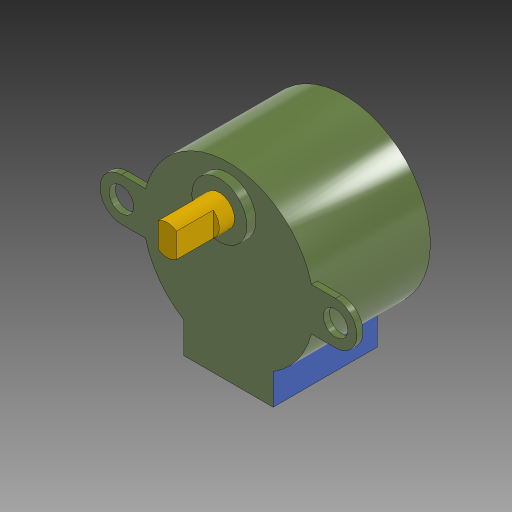
# Autodesk Inventor part: StepperMotor
Saved by Autodesk Inventor 2023 (Build 270158000, 158)
## iProperties
Created: 2024-02-02
Part Number: StepperMotor
Material: Všeobecné
Document SubType Name: Modeling
Designer: matej
Mass: 12.9017 g
Surface Area: 35.146 cm^2
Volume: 12.9017 cm^3
Density: 1 g/cm^3
Appearance: Tmavě olivová
Author: matej
Autodesk Inventor part; units mm, degrees
ref_plane "YZ Plane" through (0, 0, 0) normal (1, 0, 0) x (0, 1, 0)
ref_plane "XZ Plane" through (0, 0, 0) normal (0, 1, 0) x (-1, 0, 0)
ref_plane "XY Plane" through (0, 0, 0) normal (0, 0, 1) x (1, 0, 0)
sketch "Náčrt1" plane through (0, 0, 0) normal (0, 0, 1) x (1, 0, 0)
  circle A0 centre (0, 0) radius 14
  dimension "d0" = 28
  constraints: 1 centre point, 1 coincident
  measures "d0" diameter of A0
extrude "Vysunutí1" add sketch "Náčrt1" along normal blind 19
sketch "Náčrt2" plane through (0, 0, 19) normal (0, 0, 1) x (1, 0, 0)
  circle A0 centre (17.5, 0) radius 2
  circle A1 centre (-17.5, 0) radius 2
  line L0 (-17.5, 0) -> (17.5, 0) construction
  line L1 (-17.5, -3.5) -> (17.5, -3.5)
  line L2 (17.5, 3.5) -> (-17.5, 3.5)
  arc A2 (-17.5, 3.5) -> (-17.5, -3.5) centre (-17.5, 0) ccw
  arc A3 (17.5, -3.5) -> (17.5, 3.5) centre (17.5, 0) ccw
  point P0 (0, 0)
  point P1 (0, 0)
  dimension "d3" = 4
  dimension "d4" = 4
  dimension "d5" = 35
  dimension "d9" = 17.5
  dimension "d10" = 7
  constraints: 8 end point, 4 centre point, 4 point on circle, 4 tangent, 1 horizontal, 1 midpoint, 1 parallel
  measures "d3" diameter of A0
  measures "d4" diameter of A1
  measures "d5" distance of L0.end L0.start
  measures "d9" distance of point (0, 0) L0.end
  measures "d10" diameter of A3
extrude "Vysunutí2" add sketch "Náčrt2" against normal blind 1
sketch "Náčrt3" plane through (0, 0, 19) normal (0, 0, 1) x (1, 0, 0)
  circle A0 centre (0, 8) radius 4.5
  point P0 (0, 0)
  dimension "d13" = 9
  dimension "d14" = 8
  constraints: 1 centre point
  measures "d13" diameter of A0
  measures "d14" distance of point (0, 0) A0.centre
extrude "Vysunutí3" add sketch "Náčrt3" along normal blind 1.5
sketch "Náčrt4" plane through (0, 8, 20.5) normal (0, 0, 1) x (1, 0, 0)
  circle A0 centre (0, 0) radius 2.5
  point P0 (0, -8)
  dimension "d17" = 5
  constraints: 1 centre point
  measures "d17" diameter of A0
extrude "Vysunutí4" add sketch "Náčrt4" along normal blind 8.5
sketch "Náčrt5" plane through (0, 8, 29) normal (0, 0, 1) x (1, 0, 0)
  line L0 (-1.5, -2.5) -> (1.5, -2.5)
  line L1 (1.5, -2.5) -> (1.5, 2.5)
  line L2 (1.5, 2.5) -> (-1.5, 2.5)
  line L3 (-1.5, 2.5) -> (-1.5, -2.5)
  line L4 (-1.5, -2.5) -> (1.5, 2.5) construction
  line L5 (1.5, -2.5) -> (-1.5, 2.5) construction
  line L6 (-3, -3) -> (3, -3)
  line L7 (3, -3) -> (3, 3)
  line L8 (3, 3) -> (-3, 3)
  line L9 (-3, 3) -> (-3, -3)
  line L10 (-3, -3) -> (3, 3) construction
  line L11 (3, -3) -> (-3, 3) construction
  point P0 (0, -8)
  point P1 (0, 0)
  point P2 (0, 0)
  dimension "d20" = 3
  dimension "d21" = 5
  dimension "d22" = 6
  dimension "d23" = 6
  constraints: 24 end point, 5 midpoint, 4 parallel, 2 horizontal, 2 perpendicular
  measures "d20" distance of L2.end L1.end
  measures "d21" distance of L1.end L0.end
  measures "d22" distance of L8.end L7.end
  measures "d23" distance of L7.end L6.end
extrude "Vysunutí5" cut sketch "Náčrt5" against normal blind 6
sketch "Náčrt6" plane through (0, 0, 19) normal (0, 0, 1) x (1, 0, 0)
  line L0 (-7.3, 17) -> (7.3, 17)
  line L1 (7.3, 17) -> (7.3, -17)
  line L2 (7.3, -17) -> (-7.3, -17)
  line L3 (-7.3, -17) -> (-7.3, 17)
  line L4 (-7.3, 17) -> (7.3, -17) construction
  line L5 (7.3, 17) -> (-7.3, -17) construction
  line L6 (-7.3, -8.0625) -> (7.3, -8.0625)
  point P0 (0, 0)
  dimension "d26" = 14.6
  dimension "d27" = 34
  constraints: 14 end point, 2 midpoint, 2 parallel, 2 perpendicular, 2 point on line, 1 horizontal
  measures "d26" distance of L1.end L2.end
  measures "d27" distance of L0.end L1.end
extrude "Vysunutí6" add sketch "Náčrt6" against normal blind 17 contours L6 L1 L2 L3
